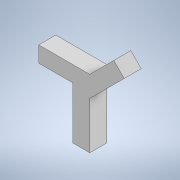
# Autodesk Inventor part: example01
Saved by Autodesk Inventor 2021.1 (Build 251245000, 245)
## iProperties
Created: 2020-09-23
Part Number: example01
Material: Generic
Document SubType Name: Modeling
Designer: robst
Density: 1 g/cm^3
Appearance: Default
Author: robst
Autodesk Inventor part; units mm, degrees
ref_plane "YZ Plane" through (0, 0, 0) normal (1, 0, 0) x (0, 1, 0)
ref_plane "XZ Plane" through (0, 0, 0) normal (0, 1, 0) x (-1, 0, 0)
ref_plane "XY Plane" through (0, 0, 0) normal (0, 0, 1) x (1, 0, 0)
sketch "Sketch1" plane through (0, 0, 0) normal (0, 1, 0) x (-1, 0, 0)
  line L0 (-12.7, 12.7) -> (-12.7, -12.7)
  line L1 (-12.7, -12.7) -> (12.7, -12.7)
  line L2 (12.7, -12.7) -> (12.7, 12.7)
  line L3 (12.7, 12.7) -> (-12.7, 12.7)
  line L4 (-12.7, 12.7) -> (12.7, -12.7) construction
  line L5 (-12.7, -12.7) -> (12.7, 12.7) construction
  point P0 (0, 0)
  dimension "d0" = 25.4
  constraints: 12 end point, 2 midpoint, 2 parallel, 2 perpendicular, 1 vertical
  measures "d0" distance of L1.end L0.end
extrude "Extrusion1" add sketch "Sketch1" along normal blind 101.6
sketch "Sketch3" plane through (-12.7, 0, -12.7) normal (-1, 0, 0) x (0, 0, 1)
  line L0 (25.4, 101.6) -> (0, 101.6) projected
  line L1 (0, 101.6) -> (25.4, 101.6)
  line L2 (25.4, 101.6) -> (25.4, 77.8642)
  line L3 (25.4, 77.8642) -> (0, 77.8642)
  line L4 (0, 77.8642) -> (0, 101.6)
  point P0 (12.7, 0)
  constraints: 8 end point, 2 parallel, 1 horizontal, 1 perpendicular
extrude "Extrusion3" add sketch "Sketch3" along normal blind 50.8
sketch "Sketch4" plane through (-12.7, 0, 12.7) normal (0, 0, 1) x (1, 0, 0)
  line L0 (25.4, 0) -> (25.4, 101.6) projected
  line L1 (25.4, 101.6) -> (61.321, 137.521)
  line L2 (25.4, 101.6) -> (76.2, 101.6) construction
  line L3 (61.321, 137.521) -> (76.8907, 121.9514)
  line L4 (76.8907, 121.9514) -> (25.4, 70.4607)
  point P0 (12.7, 0)
  dimension "d7" = 50.8
  dimension "d8" = 45
  constraints: 8 end point, 2 perpendicular, 1 equal length, 1 horizontal, 1 point on line
  measures "d7" distance of L0.end L1.end
  measures "d8" angle of L2 L1
extrude "Extrusion4" add sketch "Sketch4" against normal blind 25.4
body "Solid1"
